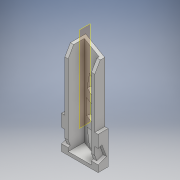
# Autodesk Inventor part: k2_t
Saved by Autodesk Inventor 2017 (Build 210142000, 142)
## iProperties
Created: 2017-02-09
Part Number: k2_t
Material: Generic
Document SubType Name: Modeling
Designer: herman
Density: 1 g/cm^3
Appearance: Default
Author: herman
Autodesk Inventor part; units mm, degrees
ref_plane "YZ Plane" through (0, 0, 0) normal (1, 0, 0) x (0, 1, 0)
ref_plane "XZ Plane" through (0, 0, 0) normal (0, 1, 0) x (-1, 0, 0)
ref_plane "XY Plane" through (0, 0, 0) normal (0, 0, 1) x (1, 0, 0)
sketch "Sketch1" plane through (0, 0, 0) normal (0, 0, 1) x (1, 0, 0)
  line L0 (-8.4365, 10.4464) -> (-8.4365, -8.3808)
  line L1 (-8.4365, -8.3808) -> (18.5635, -8.3808)
  line L2 (18.5635, -8.3808) -> (18.5635, 0.6192)
  line L3 (18.5635, 0.6192) -> (-8.4365, 10.4464)
  point P0 (0, 0)
  dimension "d0" = 9
  dimension "d2" = 110
  dimension "d30" = 27
  constraints: 8 end point, 2 perpendicular, 1 vertical
  measures "d0" distance of L1.end L2.end
  measures "d2" angle of L3 L2
  measures "d30" distance of L0.end L1.end
extrude "Extrusion1" add sketch "Sketch1" along normal blind 100
sketch "Sketch2" plane through (-8.4365, 10.4464, 100) normal (0.3420201, 0.9396926, 0) x (0.9396926, -0.3420201, 0)
  line L0 (7.4677, 59.9801) -> (21.4677, 59.9801)
  line L1 (21.4677, 59.9801) -> (21.4677, 73.9801)
  line L2 (21.4677, 73.9801) -> (7.4677, 73.9801)
  line L3 (7.4677, 73.9801) -> (7.4677, 59.9801)
  line L4 (0, 100) -> (0, 0) projected
  line L5 (28.7328, 100) -> (0, 100) projected
  line L6 (28.7328, 100) -> (28.7328, 0) projected
  line L7 (21.4677, 66.9801) -> (93.4677, 66.9801) construction
  line L8 (23.9211, 48.3451) -> (93.4677, 66.9801) construction
  line L9 (12.2098, 37.9602) -> (25.7328, 41.5836)
  line L10 (25.7328, 41.5836) -> (22.1093, 55.1066)
  line L11 (22.1093, 55.1066) -> (8.5864, 51.4831)
  line L12 (8.5864, 51.4831) -> (12.2098, 37.9602)
  line L13 (8.5864, 82.477) -> (22.1093, 78.8536)
  line L14 (22.1093, 78.8536) -> (25.7328, 92.3765)
  line L15 (25.7328, 92.3765) -> (12.2098, 96)
  line L16 (12.2098, 96) -> (8.5864, 82.477)
  point P0 (11.5006, 100)
  point P1 (23.9211, 85.6151)
  dimension "d5" = 14
  dimension "d6" = 14
  dimension "d9" = 72
  dimension "d12" = 15
  dimension "d16" = 15
  dimension "d19" = 4
  dimension "d46" = 3
  constraints: 28 end point, 2 horizontal, 2 parallel, 1 coincident, 1 midpoint, 1 perpendicular, 21 other
  measures "d5" distance of L1.end L2.end
  measures "d6" distance of L0.end L1.end
  measures "d9" distance of L7.start L7.end
  measures "d19" distance from line of L5 L15.end
  measures "d46" distance from line of L6 L9.end
sketch "Sketch3" plane through (18.5635, -8.3808, 0) normal (1, 0, 0) x (0, 0, -1)
  line L0 (0, 9) -> (-100, 9) projected
  line L1 (0, 9) -> (-30, 9)
  line L2 (-30, 9) -> (-30, 0)
  line L3 (0, 0) -> (0, 9)
  line L4 (0, 9) -> (0, 18.8272) projected
  line L5 (0, 9) -> (0, 0)
  line L6 (0, 0) -> (-6.123, 0)
  line L7 (-18.8931, 0) -> (-30, 0)
  line L8 (0, 0) -> (-100, 0) projected
  line L9 (-18.8931, 0) -> (-20.1355, 3.4133)
  line L10 (-20.1355, 3.4133) -> (-8.8592, 7.5175)
  line L11 (-8.8592, 7.5175) -> (-6.123, 0)
  point P0 (0, 8.3808)
  dimension "d26" = 30
  dimension "d52" = 12
  dimension "d53" = 110
  dimension "d60" = 8
  constraints: 18 end point, 4 perpendicular, 2 horizontal, 1 parallel, 1 point on line
  measures "d26" distance of L0.start L1.end
  measures "d52" distance of L9.end L10.end
  measures "d53" angle of L11 L6
  measures "d60" distance of L6.end L10.end
ref_plane "Work Plane1" through (5.0635, -8.3808, 100) normal (1, 0, 0) x (0, 0, -1)
sketch "Sketch4" plane through (-8.4365, -8.3808, 100) normal (-1, 0, 0) x (0, 0, 1)
  line L0 (-100, 18.8272) -> (0, 18.8272) projected
  line L1 (0, 18.8272) -> (0, 0) projected
  line L2 (-100, 0) -> (0, 0) projected
  line L3 (-15.9164, 18.8272) -> (0, 18.8272)
  line L4 (0, 0) -> (-24.5767, 0)
  line L5 (-100, 0) -> (0, 0) projected
  line L6 (0, 9) -> (0, 18.8272) projected
  line L7 (0, 0) -> (0, 9) projected
  line L8 (0, 18.8272) -> (0, 0)
  line L9 (-24.5767, 0) -> (-15.9164, 5)
  line L10 (-15.9164, 5) -> (-15.9164, 18.8272)
  line L11 (-70, 0) -> (-83.5767, 0) projected
  point P0 (-100, 8.3808)
  dimension "d33" = 10
  dimension "d34" = 30
  dimension "d35" = 59
  constraints: 10 end point, 2 point on line, 1 collinear, 1 perpendicular, 1 vertical
  measures "d33" distance of L4.end L9.end
  measures "d34" angle of L2 L9
  measures "d35" distance of L4.end L11.end
thicken "Thicken1" operation intersect thickness 3 both sides no extend neighbours no toward (-1, 0, 0) faces at (18.5635, -5.3808, 33.3333) (9.5635, 3.895, 33.3333) (0.5635, 0.895, 0) (-8.4365, 4.1707, 66.6667) (0.5635, 0.895, 100)
extrude "Extrusion5" cut sketch "Sketch4" against normal through all
extrude "Extrusion6" add sketch "Sketch3" along normal blind 3 contours L3 L6 L11 L10 L9 L7 L2 L0
mirror "Mirror2" about plane through (5.0635, -8.3808, 100) normal (1, 0, 0) of "Extrusion6"
extrude "Extrusion7" cut sketch "Sketch2" against normal up to next
sketch "Sketch5" plane through (18.5635, -8.3808, 18.8931) normal (1, 0, 0) x (0, 0, -1)
  line L0 (12.7701, 0) -> (0, 0) projected
  line L1 (12.7701, 0) -> (10.034, 7.5175) projected
  line L2 (12.0861, 1.8794) -> (6.9225, 0)
  line L3 (12.0861, 1.8794) -> (12.7701, 0)
  line L4 (6.9225, 0) -> (12.7701, 0)
  line L5 (15.8931, 0) -> (-56.5302, 0) projected
  point P0 (18.8931, 8.3808)
  dimension "d57" = 2
  constraints: 6 end point, 2 collinear, 2 point on line, 1 perpendicular
  measures "d57" distance of L0.start L2.start
extrude "Extrusion8" cut sketch "Sketch5" against normal through all
body "Solid1"
